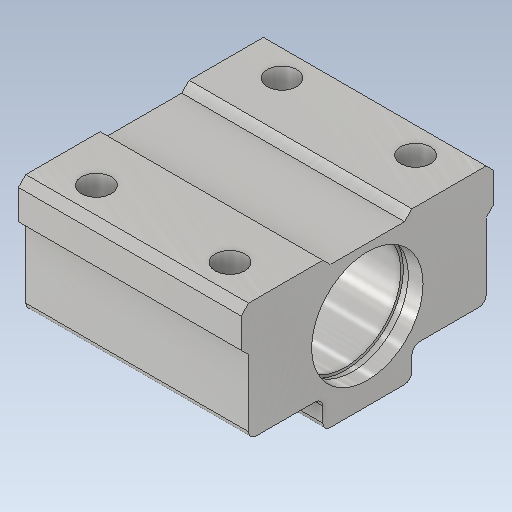
# Autodesk Inventor part: 16_obudowa łożyska
Saved by Autodesk Inventor 2020.2 (Build 242310000, 310)
## iProperties
Created: 2017-10-08
Part Number: 16_obudowa łożyska
Material: Ogólny
Document SubType Name: Modeling
Designer: Haras
Density: 1 g/cm^3
Appearance: Obrobione — aluminium
Author: Haras
Autodesk Inventor part; units mm, degrees
ref_plane "YZ Plane" through (0, 0, 0) normal (1, 0, 0) x (0, 1, 0)
sketch "Szkic1" plane through (0, 0, 0) normal (1, 0, 0) x (0, 1, 0)
  line L0 (0, 17) -> (-6, 17)
  line L1 (-6, 17) -> (-6, 16)
  line L2 (-6, 16) -> (-16, 16)
  line L3 (-16, 16) -> (-16, 6)
  line L4 (-16, 6) -> (-20, 6)
  line L5 (-20, 6) -> (-20, 0)
  line L6 (0, 17) -> (0, 5)
  line L7 (0, 5) -> (-1, 5)
  line L8 (-1, 5) -> (-1, 0)
  line L9 (-1, 0) -> (-20, 0) construction
  line L10 (0, -17) -> (-6, -17)
  line L11 (-6, -17) -> (-6, -16)
  line L12 (-6, -16) -> (-16, -16)
  line L13 (-16, -16) -> (-16, -6)
  line L14 (-16, -6) -> (-20, -6)
  line L15 (-20, -6) -> (-20, 0)
  line L16 (0, -17) -> (0, -5)
  line L17 (0, -5) -> (-1, -5)
  line L18 (-1, -5) -> (-1, 0)
  point P0 (0, 0)
  dimension "d0" = 17
  dimension "d1" = 6
  dimension "d2" = 1
  dimension "d3" = 10
  dimension "d4" = 10
  dimension "d5" = 4
  dimension "d40" = 12
  dimension "d41" = 1
  dimension "d43" = 6
  constraints: 38 end point, 8 symmetric about line, 7 perpendicular, 2 horizontal, 1 horizontal alignment, 1 vertical
  measures "d0" distance of point (0, 0) L0.start
  measures "d1" distance of L0.start L0.end
  measures "d2" distance of L0.end L1.end
  measures "d3" distance of L1.end L2.end
  measures "d4" distance of L2.end L3.end
  measures "d5" distance of L3.end L4.end
  measures "d40" distance of L0.start L6.end
  measures "d41" distance of L6.end L7.end
  measures "d43" distance of L4.end L5.end
extrude "Wyciągnięcie proste1" add sketch "Szkic1" along normal blind 30
ref_plane "Płaszczyzna konstrukcyjna2" through (2, 0, 0) normal (-1, 0, 0) x (0, 0, 1)
ref_plane "Płaszczyzna konstrukcyjna3" through (15, 0, 0) normal (-1, 0, 0) x (0, 0, 1)
sketch "Szkic7" plane through (0, 0, 0) normal (-1, 0, 0) x (0, 0, 1)
  line L0 (6, -20) -> (-6, -20) projected
  point P0 (0, 0)
  point P1 (0, -9.5)
  dimension "d44" = 10.5
  constraints: 1 vertical alignment
  measures "d44" distance from line of L0 point (0, -9.5)
hole "Otwór3" at (0, -9.5, 0) direction (1, 0, 0) diameter 15 end through all
sketch "Szkic8" plane through (2, 0, 0) normal (-1, 0, 0) x (0, 0, 1)
  circle A0 centre (0, -9.5) radius 7.5 projected
  circle A1 centre (0, -9.5) radius 7.85
  point P0 (0, 0)
  dimension "d52" = 15.7
  constraints: 1 centre point, 1 coincident
  measures "d52" diameter of A1
extrude "Wyciągnięcie proste4" cut sketch "Szkic8" against normal blind 1
mirror "Odbij2" about plane through (15, 0, 0) normal (-1, 0, 0) of "Wyciągnięcie proste4"
sketch "Szkic9" plane through (0, 0, 17) normal (0, 1, 0) x (1, 0, 0)
  line L0 (0, 0) -> (30, 0) projected
  line L1 (30, 12) -> (30, 0) projected
  point P0 (0, 17)
  point P1 (24, 29.5)
  point P2 (24, 4.5)
  point P3 (6, 4.5)
  point P4 (6, 29.5)
  dimension "d55" = 18
  dimension "d56" = 25
  dimension "d57" = 4.5
  dimension "d58" = 6
  constraints: 2 horizontal alignment, 2 vertical alignment
  measures "d55" distance of point (6, 4.5) point (24, 4.5)
  measures "d56" distance of point (24, 4.5) point (24, 29.5)
  measures "d57" distance from line of L0 point (24, 4.5)
  measures "d58" distance from line of L1 point (24, 4.5)
chamfer "Faza2" distance 1 angle 45 6 edges at (15, 0, 5) (15, 0, -5) (15, 0, 17) (15, 0, -17) (15, -6, -17) (15, -6, 17)
fillet "Zaokrąglenie2" radius 1 6 edges at (15, -16, 16) (15, -20, 6) (15, -20, -6) (15, -16, -16) (15, -16, 6) (15, -16, -6)
hole "Otwór5" at (24, 0, -12.5) at (24, 0, 12.5) at (6, 0, 12.5) at (6, 0, -12.5) direction (0, -1, 0) diameter 4 end through all
chamfer "Faza3" distance 0.5 angle 45 4 edges at (24, -16, 10.5) (6, -16, 10.5) (24, -16, -14.5) (6, -16, -14.5)
